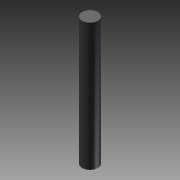
# Autodesk Inventor part: SHPSNA5_1
Saved by Autodesk Inventor 2015 SP1 (Build 190203100, 203)
## iProperties
Category: PARTsolutions
Company: MISUMI
Created: 2015-01-26
Part Number: SHPSNA5_1
Catalog Web Link: www.cadenas.de
Description: SHPSNA_1-Hinges with Slotted Holes
Vendor: MISUMI
Document SubType Name: Modeling
Designer: PARTuser1
Manufacturer: MISUMI
Mass: 0.805033 g
Surface Area: 6.83296 cm^2
Volume: 0.805033 cm^3
Density: 1 g/cm^3
Material: Generic
Appearance: PSOLRGB-192-192-192
PSOL_IDENT_0: {\\10.0.0.236\data_v8\23d-libs\misumi\metric\44_handles_hinges\shpsna_1.prj},162 {VTYP=3D},{NB=SHPSN
PSOL_IDENT_1: A5_1},{LINA=SHPSNA5_1},{NN=SHPSNA_1},{DATE=14.11.2014 09:15:25},{GEOMDATE=20.01.2009 08:56:00},{VERS
PSOL_IDENT_2: ION=},{LINEID=10},{LINESUBID=-1},{WBVAR=}  {NB=SHPSNA5_1},{LINA=SHPSNA5_1},{KT=DUMMY},{PN=SHPSNA5},{
PSOL_IDENT_3: TYPE=SHPSNA},{MAT=304 Stainless Steel},{NO=5},{AL1=9},{AL2=88},{MASS=43},{L=41},{W=36},{K=8},{P=25},
PSOL_IDENT_4: {J=7.5},{S=21},{N=5.5},{Z=5.5x6.5},{Z1=5.5},{Z2=6.5},{T=2},{E=4.6},{R=4.6},{CR=4},{D=5}
SUPPLIER: MISUMI
ARTICLENO: SHPSNA5_1
BOMINFO: SHPSNA5_1
CREATOR: CADENAS GmbH
Title: SHPSNA5_1
Author: Cadenas PARTsolutions
Comments: Hinges with Slotted Holes
Autodesk Inventor part; units mm, degrees
sketch "Sketch_1" plane through (0, 0, 0) normal (0, 0, 1) x (1, 0, 0)
  circle A0 centre (0, 0) radius 2.5
  constraints: 1 centre point
extrude "Extrusion1" add sketch "Sketch_1" along normal blind 41
ref_plane "1_to_2_XY" through (0, 0, 20.5) normal (0, 0, 1) x (1, 0, 0)
ref_plane "1_to_2_YZ" through (0, 0, 20.5) normal (1, 0, 0) x (0, 1, 0)
ref_plane "1_to_2_ZX" through (0, 0, 20.5) normal (0, 1, 0) x (0, 0, 1)
ref_plane "1_to_3_XY" through (0, 0, 20.5) normal (0, 0, 1) x (1, 0, 0)
ref_plane "1_to_3_YZ" through (0, 0, 20.5) normal (1, 0, 0) x (0, 1, 0)
ref_plane "1_to_3_ZX" through (0, 0, 20.5) normal (0, 1, 0) x (0, 0, 1)
body "Solid1"
